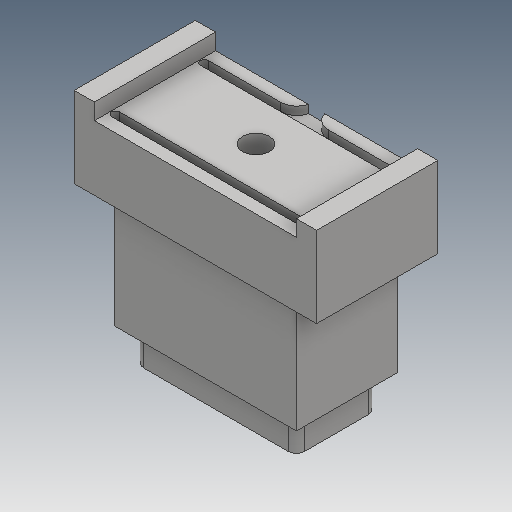
# Autodesk Inventor part: 10x20mm_Cuvette_Top
Saved by Autodesk Inventor 2019 (Build 230136000, 136)
## iProperties
Created: 2018-07-25
Part Number: 10x20mm_Cuvette_Top
Material: Generic
Document SubType Name: Modeling
Designer: voigt
Density: 1 g/cm^3
Appearance: Default
Author: voigt
Autodesk Inventor part; units mm, degrees
ref_plane "YZ Plane" through (0, 0, 0) normal (1, 0, 0) x (0, 1, 0)
ref_plane "XZ Plane" through (0, 0, 0) normal (0, 1, 0) x (-1, 0, 0)
ref_plane "XY Plane" through (0, 0, 0) normal (0, 0, 1) x (1, 0, 0)
sketch "Sketch1" plane through (0, 0, 0) normal (0, 0, 1) x (1, 0, 0)
  line L0 (0, 10.5) -> (0, -10.5) construction
  line L1 (-21, 0) -> (21, 0) construction
  line L2 (-15, 7.5) -> (15, 7.5)
  line L3 (15, 7.5) -> (15, -7.5)
  line L4 (15, -7.5) -> (-15, -7.5)
  line L5 (-15, -7.5) -> (-15, 7.5)
  point P0 (0, 0)
  dimension "d0" = 15
  dimension "d1" = 30
  constraints: 8 end point, 2 parallel, 1 horizontal, 1 perpendicular, 2 other
  measures "d0" distance of L2.end L3.end
  measures "d1" distance of L2.start L2.end
extrude "Extrusion1" add sketch "Sketch1" along normal blind 10
sketch "Sketch2" plane through (0, 0, 0) normal (0, 0, -1) x (-1, 0, 0)
  line L0 (15, 7.5) -> (-15, 7.5) construction
  line L1 (-15, 7.5) -> (-15, -7.5) construction
  line L2 (-15, -7.5) -> (15, -7.5) construction
  line L3 (15, -7.5) -> (15, 7.5) construction
  line L4 (0, -10.5) -> (0, 10.5) construction
  line L5 (11.25, -6.25) -> (-11.25, -6.25)
  line L6 (-11.25, -6.25) -> (-11.25, 6.25)
  line L7 (-11.25, 6.25) -> (11.25, 6.25)
  line L8 (11.25, 6.25) -> (11.25, -6.25)
  line L9 (-21, 0) -> (21, 0) construction
  point P0 (0, 0)
  point P1 (-4.7643, 7.5)
  dimension "d32" = 12.5
  dimension "d33" = 22.5
  constraints: 8 end point, 2 parallel, 1 horizontal, 1 perpendicular, 1 point on line, 2 other
  measures "d32" distance between parallel lines of L7 L5
  measures "d33" distance between parallel lines of L6 L8
extrude "Extrusion2" add sketch "Sketch2" along normal blind 14
sketch "Sketch3" plane through (-15, 7.5, 10) normal (0, 1, 0) x (1, 0, 0)
  line L0 (0, 10) -> (30, 10) construction
  line L1 (0, 10) -> (0, 0) construction
  line L2 (30, 0) -> (0, 0) construction
  line L3 (30, 10) -> (30, 0) construction
  line L4 (0, 0) -> (30, 0) projected
  line L5 (27.5, 0) -> (2.5, 0)
  line L6 (2.5, 0) -> (2.5, 2)
  line L7 (2.5, 2) -> (27.5, 2)
  line L8 (27.5, 2) -> (27.5, 0)
  line L9 (15, 28.8) -> (15, -4.8) construction
  point P0 (15, 10)
  dimension "d7" = 2
  dimension "d8" = 25
  constraints: 8 end point, 2 parallel, 1 horizontal, 1 perpendicular, 1 point on line, 1 other
  measures "d7" distance between parallel lines of L2 L7
  measures "d8" distance between parallel lines of L6 L8
extrude "Extrusion3" cut sketch "Sketch3" against normal up to next
sketch "Sketch4" plane through (0, 0, -14) normal (0, 0, -1) x (-1, 0, 0)
  line L0 (0, -10.5) -> (0, 10.5) construction
  line L1 (-21, 0) -> (21, 0) construction
  line L2 (11.25, 7.5) -> (-11.25, 7.5) construction
  line L3 (-11.25, 7.5) -> (-11.25, -7.5) construction
  line L4 (-11.25, -7.5) -> (11.25, -7.5) construction
  line L5 (11.25, -7.5) -> (11.25, 7.5) construction
  line L6 (-9.95, -4.95) -> (9.95, -4.95)
  line L7 (9.95, -4.95) -> (9.95, 4.95)
  line L8 (9.95, 4.95) -> (-9.95, 4.95)
  line L9 (-9.95, 4.95) -> (-9.95, -4.95)
  point P0 (0, 0)
  dimension "d11" = 19.9
  dimension "d12" = 9.9
  constraints: 8 end point, 2 parallel, 1 horizontal, 1 perpendicular, 2 other
  measures "d11" distance of L6.start L6.end
  measures "d12" distance between parallel lines of L8 L6
extrude "Extrusion4" add sketch "Sketch4" along normal blind 4
sketch "Sketch5" plane through (-12.5, 7.5, 8) normal (0, 0, 1) x (1, 0, 0)
  point P0 (12.5, -7.5)
  point P1 (12.5, -7.5)
  constraints: 1 coincident
hole "Hole1" at (0, 0, 8) direction (0, 0, -1) diameter 3.3 end through all
fillet "Fillet1" radius 1 4 edges at (9.95, -4.95, -16) (9.95, 4.95, -16) (-9.95, 4.95, -16) (-9.95, -4.95, -16)
sketch "Sketch7" plane through (0, 0, 0) normal (0, 0, -1) x (-1, 0, 0)
  line L0 (-11.25, -6.25) -> (-11.25, 6.25) construction
  line L1 (-11.25, 6.25) -> (11.25, 6.25) construction
  line L2 (11.25, 6.25) -> (11.25, -6.25) construction
  line L3 (11.25, -6.25) -> (-11.25, -6.25) construction
  line L4 (15, 7.5) -> (-15, 7.5) construction
  line L5 (-15, 7.5) -> (-15, -7.5) construction
  line L6 (-15, -7.5) -> (15, -7.5) construction
  line L7 (15, -7.5) -> (15, 7.5) construction
  line L8 (-21, 0) -> (21, 0) construction
  point P0 (0, 0)
  point P1 (-11.875, -5.5)
  point P2 (-11.875, 5.5)
  point P3 (11.875, -5.5)
  point P4 (11.875, 5.5)
  dimension "d34" = 0.625
  dimension "d35" = 5.5
  dimension "d36" = 0.625
  dimension "d37" = 5.5
  dimension "d38" = 0.625
  dimension "d39" = 0.625
  dimension "d40" = 5.5
  dimension "d41" = 5.5
  measures "d34" distance from line of L0 point (-11.875, -5.5)
  measures "d35" distance from line of L8 point (-11.875, -5.5)
  measures "d36" distance from line of L0 point (-11.875, 5.5)
  measures "d37" distance from line of L8 point (-11.875, 5.5)
  measures "d38" distance from line of L2 point (11.875, 5.5)
  measures "d39" distance from line of L2 point (11.875, -5.5)
  measures "d40" distance from line of L8 point (11.875, -5.5)
  measures "d41" distance from line of L8 point (11.875, 5.5)
hole "Hole3" at (11.875, -5.5, 0) at (11.875, 5.5, 0) at (-11.875, -5.5, 0) at (-11.875, 5.5, 0) direction (0, 0, 1) diameter 1 end through all
sketch "Sketch8" plane through (-12.5, 7.5, 8) normal (0, 0, 1) x (1, 0, 0)
  circle A0 centre (0.625, -13) radius 0.5 construction
  circle A1 centre (24.375, -13) radius 0.5 construction
  circle A2 centre (24.375, -2) radius 0.5 construction
  circle A3 centre (0.625, -2) radius 0.5 construction
  circle A4 centre (12.5, -7.5) radius 1.65 construction
  line L0 (25, -15) -> (0, -15) construction
  line L1 (25, 0) -> (25, -15) construction
  line L2 (0, 0) -> (25, 0) construction
  line L3 (0, 0) -> (0, -15) construction
  line L4 (0.625, -1.5) -> (24.375, -1.5)
  line L5 (24.375, -1.5) -> (24.375, -2.5)
  line L6 (24.375, -2.5) -> (0.625, -2.5)
  line L7 (0.625, -2.5) -> (0.625, -1.5)
  circle A5 centre (0.625, -13) radius 0.5 projected
  line L8 (0.625, -12.5) -> (24.3681, -12.5)
  line L9 (24.3681, -12.5) -> (24.3681, -13.5)
  line L10 (24.3681, -13.5) -> (0.625, -13.5)
  line L11 (0.625, -13.5) -> (0.625, -12.5)
  point P0 (12.5, -7.5)
  dimension "d49" = 1
  dimension "d50" = 0.625
  dimension "d51" = 1
  dimension "d52" = 0.625
  constraints: 16 end point, 4 parallel, 4 vertical alignment, 2 horizontal, 2 perpendicular, 6 other
  measures "d49" distance between parallel lines of L6 L4
  measures "d50" distance between parallel lines of L3 L7
  measures "d51" distance between parallel lines of L10 L8
  measures "d52" distance between parallel lines of L3 L11
extrude "Extrusion5" cut sketch "Sketch8" against normal blind 1 contours L4 L5 L6 L7 | A5 L11 | A5 L8 L9 L10 picked at (0.7752, -12.9277)
fillet "Fillet2" radius 2 4 edges at (-11.375, 5.5, 7) (11.375, 5.5, 7) (11.375, -5.5, 7) (-11.375, -5.5, 7)
sketch "Sketch9" plane through (-12.5, 7.5, 8) normal (0, 0, 1) x (1, 0, 0)
  line L0 (24.3681, -13.5) -> (0.6319, -13.5) construction
  arc A0 (0.625, -12.5) -> (0.6319, -13.5) centre (0.625, -13) ccw construction
  line L1 (0.625, -12.5) -> (24.3681, -12.5) construction
  line L2 (24.3681, -12.5) -> (24.3681, -12.5) construction
  arc A1 (24.3681, -13.5) -> (24.3681, -12.5) centre (24.375, -13) ccw construction
  line L3 (24.375, -2.5) -> (0.625, -2.5) construction
  arc A2 (0.625, -1.5) -> (0.625, -2.5) centre (0.625, -2) ccw construction
  line L4 (0.625, -1.5) -> (24.375, -1.5) construction
  arc A3 (24.375, -2.5) -> (24.375, -1.5) centre (24.375, -2) ccw construction
  circle A4 centre (12.5, -7.5) radius 1.65 construction
  line L5 (25, -15) -> (0, -15) construction
  line L6 (25, 0) -> (25, -15) construction
  line L7 (0, 0) -> (25, 0) construction
  line L8 (0, 0) -> (0, -15) construction
  line L9 (12.5, 3) -> (12.5, -18) construction
  line L10 (0.625, -1.5) -> (24.375, -1.5) projected
  line L11 (0, 0) -> (25, 0) projected
  line L12 (13.5, -1.5) -> (11.5, -1.5)
  line L13 (11.5, -1.5) -> (11.5, 0)
  line L14 (11.5, 0) -> (13.5, 0)
  line L15 (13.5, 0) -> (13.5, -1.5)
  point P0 (12.5, -7.5)
  dimension "d56" = 2
  constraints: 8 end point, 2 parallel, 2 point on line, 1 horizontal, 1 perpendicular, 1 other
  measures "d56" distance between parallel lines of L13 L15
extrude "Extrusion6" cut sketch "Sketch9" against normal up to surface (1 mm away)
fillet "Fillet3" radius 2 2 edges at (-1, 6, 7.5) (1, 6, 7.5)
body "Solid1"
